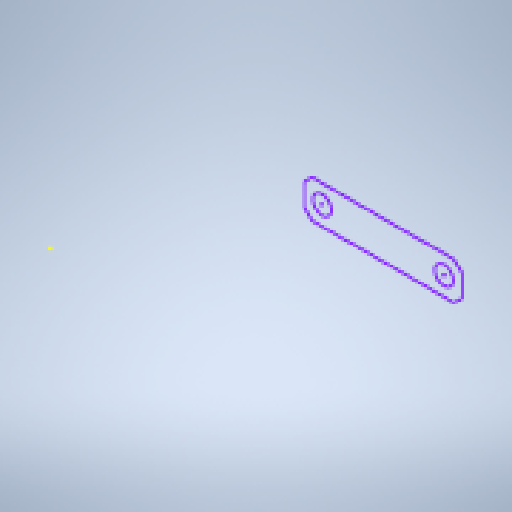
# Autodesk Inventor part: suporte_mancal
Saved by Autodesk Inventor 2023 (Build 270158000, 158)
## iProperties
Created: 2022-10-25
Part Number: suporte_mancal
Material: Generic
Document SubType Name: Modeling
Designer: klebe
Density: 1 g/cm^3
Appearance: Default
Author: klebe
Autodesk Inventor part; units mm, degrees
ref_plane "YZ Plane" through (0, 0, 0) normal (1, 0, 0) x (0, 1, 0)
ref_plane "XZ Plane" through (0, 0, 0) normal (0, 1, 0) x (-1, 0, 0)
ref_plane "XY Plane" through (0, 0, 0) normal (0, 0, 1) x (1, 0, 0)
sketch "Sketch1" plane through (0, 0, 0) normal (0, 0, 1) x (1, 0, 0)
  circle A0 centre (167.326, 74.0027) radius 4
  line L0 (171.576, 66.0777) -> (171.576, 66.0027)
  line L1 (174.826, 69.3277) -> (171.576, 66.0777)
  line L2 (174.826, 78.6777) -> (174.826, 69.3277)
  line L3 (171.576, 81.9277) -> (174.826, 78.6777)
  line L4 (171.576, 81.9277) -> (171.576, 82.0027)
  line L5 (111.076, 81.9277) -> (111.076, 82.0027)
  line L6 (107.826, 78.6777) -> (111.076, 81.9277)
  line L7 (107.826, 78.6777) -> (107.826, 69.3277)
  line L8 (111.076, 66.0777) -> (107.826, 69.3277)
  line L9 (111.076, 66.0777) -> (111.076, 66.0027)
  circle A1 centre (115.326, 74.0027) radius 4
  line L10 (171.576, 82.0027) -> (111.076, 82.0027)
  line L11 (111.076, 66.0027) -> (171.576, 66.0027)
  point P0 (0, 0)
  constraints: 24 end point, 2 centre point, 1 horizontal, 1 parallel
extrude "Extrusion1" add sketch "Sketch1" along normal blind 4
body "Solid1"
